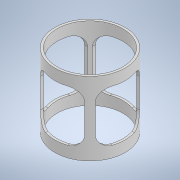
# Autodesk Inventor part: Khay đựng cốc
Saved by Autodesk Inventor 2020 (Build 240168000, 168)
## iProperties
Created: 2022-04-01
Part Number: Khay đựng cốc
Material: Generic
Document SubType Name: Modeling
Designer: PC
Density: 1 g/cm^3
Appearance: Default
Author: PC
Autodesk Inventor part; units mm, degrees
ref_plane "YZ Plane" through (0, 0, 0) normal (1, 0, 0) x (0, 1, 0)
ref_plane "XZ Plane" through (0, 0, 0) normal (0, 1, 0) x (-1, 0, 0)
ref_plane "XY Plane" through (0, 0, 0) normal (0, 0, 1) x (1, 0, 0)
sketch "Sketch1" plane through (0, 0, 0) normal (0, 1, 0) x (-1, 0, 0)
  circle A0 centre (0, 0) radius 48
  dimension "d0" = 96
  constraints: 1 centre point, 1 coincident
  measures "d0" diameter of A0
extrude "Extrusion1" add sketch "Sketch1" along normal blind 100
sketch "Sketch2" plane through (0, 100, 0) normal (0, 1, 0) x (1, 0, 0)
  circle A0 centre (0, 0) radius 45
  dimension "d3" = 90
  constraints: 1 centre point, 1 coincident
  measures "d3" diameter of A0
extrude "Extrusion2" cut sketch "Sketch2" against normal blind 100
sketch "Sketch3" plane through (0, 0, 0) normal (0, 0, 1) x (1, 0, 0)
  line L0 (-15, 85) -> (15, 85)
  line L1 (30, 70) -> (30, 30)
  line L2 (15, 15) -> (-15, 15)
  line L3 (-30, 30) -> (-30, 70)
  line L4 (-30, 85) -> (30, 15) construction
  line L5 (30, 85) -> (-30, 15) construction
  arc A0 (30, 70) -> (15, 85) centre (15, 70) ccw
  arc A1 (-15, 85) -> (-30, 70) centre (-15, 70) ccw
  arc A2 (-30, 30) -> (-15, 15) centre (-15, 30) ccw
  arc A3 (15, 15) -> (30, 30) centre (15, 30) ccw
  point P0 (0, 0)
  point P1 (0, 50)
  dimension "d6" = 60
  dimension "d7" = 70
  dimension "d8" = 15
  constraints: 12 end point, 8 point on circle, 8 point on line, 8 tangent, 4 centre point, 3 equal radius, 2 midpoint, 2 parallel, 1 horizontal, 1 perpendicular
  measures "d6" distance of L4.end L5.end
  measures "d7" distance of L5.start L4.end
  measures "d8" radius of A0
extrude "Extrusion3" cut sketch "Sketch3" along normal blind 100
pattern_circular "Circular Pattern1" count 4 over 360 about axis through (0, 100, 0) along (0, -1, 0) of "Extrusion3"
body "Solid1"
